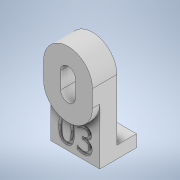
# Autodesk Inventor part: 1번부품
Saved by Autodesk Inventor 2022 (Build 260153000, 153)
## iProperties
Created: 2021-09-05
Part Number: 1번부품
Material: 일반
Document SubType Name: Modeling
Designer: 서울공업고등학교
Density: 1 g/cm^3
Appearance: 기본값
Author: 서울공업고등학교
Autodesk Inventor part; units mm, degrees
ref_plane "YZ Plane" through (0, 0, 0) normal (1, 0, 0) x (0, 1, 0)
ref_plane "XZ Plane" through (0, 0, 0) normal (0, 1, 0) x (-1, 0, 0)
ref_plane "XY Plane" through (0, 0, 0) normal (0, 0, 1) x (1, 0, 0)
sketch "스케치1" plane through (0, 0, 0) normal (0, 0, 1) x (1, 0, 0)
  line L0 (0, 0) -> (20, 0)
  line L1 (20, 0) -> (20, 40)
  line L2 (20, 40) -> (0, 40)
  line L3 (0, 40) -> (0, 0)
  line L4 (0, 13) -> (20, 13)
  line L5 (10, 30) -> (10, 23) construction
  line L6 (7, 30) -> (7, 23)
  line L7 (13, 23) -> (13, 30)
  arc A0 (13, 30) -> (7, 30) centre (10, 30) ccw
  arc A1 (7, 23) -> (13, 23) centre (10, 23) ccw
  point P0 (10, 26.5)
  dimension "d0" = 20
  dimension "d1" = 40
  dimension "d2" = 27
  dimension "d4" = 7
  dimension "d5" = 13.5
  dimension "d6" = 10
  dimension "d7" = 3
  constraints: 18 end point, 4 point on circle, 4 tangent, 3 parallel, 2 centre point, 2 perpendicular, 2 point on line, 1 horizontal, 1 midpoint, 1 vertical
  measures "d0" distance of L2.end L1.end
  measures "d1" distance of L1.end L0.end
  measures "d2" distance between parallel lines of L4 L2
  measures "d4" distance of L5.end L5.start
  measures "d5" distance from line of L2 point (10, 26.5)
  measures "d6" horizontal distance of L4.start L5.start
  measures "d7" radius of A1
extrude "돌출1" add sketch "스케치1" against normal blind 7
extrude "돌출2" add sketch "스케치1" along normal blind 3 contours L3 L2 L1 L4
fillet "모깎기1" radius 10 4 edges at (20, 40, -2) (0, 40, -2) (20, 13, 1.5) (0, 13, 1.5)
sketch "스케치2" plane through (0, 0, -7) normal (0, 0, -1) x (-1, 0, 0)
  line L0 (-20, 0) -> (-20, 23) projected
  line L1 (-20, 0) -> (0, 0) projected
  line L2 (-20, 0) -> (-20, 30) projected
  arc A0 (0, 30) -> (-20, 30) centre (-10, 30) ccw projected
  line L3 (0, 30) -> (0, 0) projected
  line L4 (0, 0) -> (-20, 0) projected
  line L5 (-13, 30) -> (-13, 23) projected
  arc A1 (-13, 23) -> (-7, 23) centre (-10, 23) ccw projected
  line L6 (-7, 23) -> (-7, 30) projected
  arc A2 (-7, 30) -> (-13, 30) centre (-10, 30) ccw projected
  line L7 (-20, 5) -> (0, 5)
  dimension "d14" = 5
  constraints: 2 end point, 2 point on line, 1 perpendicular
  measures "d14" distance between parallel lines of L1 L7
extrude "돌출3" add sketch "스케치2" along normal blind 8 contours L0 L7 L3 L1
sketch "스케치3" plane through (0, 0, 0) normal (0, 0, 1) x (1, 0, 0)
  line L0 (2.6578, 12.3276) -> (17.6998, 12.3276) construction
  line L1 (17.6998, 12.3276) -> (17.6998, 1.5834) construction
  line L2 (17.6998, 1.5834) -> (2.6578, 1.5834) construction
  line L3 (2.6578, 1.5834) -> (2.6578, 12.3276) construction
  spline S0 degree 2 poles (9.6108, 7.1169) (9.6108, 4.4265) (8.0468, 1.9062) (6.4179, 1.9062) knots 0 0 0 1 2 2 2
  spline S1 degree 2 poles (6.4179, 1.9062) (4.7648, 1.9062) (3.217, 4.4751) (3.217, 7.1088) knots 0 0 0 1 2 2 2
  spline S2 degree 2 poles (3.217, 7.1088) (3.217, 9.8155) (4.781, 12.3195) (6.4179, 12.3195) knots 0 0 0 1 2 2 2
  spline S3 degree 2 poles (6.4179, 12.3195) (8.063, 12.3195) (9.6108, 9.7263) (9.6108, 7.1169) knots 0 0 0 1 2 2 2
  spline S4 degree 2 poles (7.8928, 4.0699) (8.0873, 4.5643) (8.2494, 6.0878) (8.2494, 7.1169) knots 0 0 0 1 2 2 2
  spline S5 degree 2 poles (8.2494, 7.1169) (8.2494, 8.1461) (8.0873, 9.6615) (7.8847, 10.1721) knots 0 0 0 1 2 2 2
  spline S6 degree 2 poles (7.8847, 10.1721) (7.6821, 10.6826) (6.9771, 11.2093) (6.4179, 11.2093) knots 0 0 0 1 2 2 2
  spline S7 degree 2 poles (6.4179, 11.2093) (5.8588, 11.2093) (5.1375, 10.6826) (4.9268, 10.1558) knots 0 0 0 1 2 2 2
  spline S8 degree 2 poles (4.9268, 10.1558) (4.7242, 9.6453) (4.5784, 8.0894) (4.5784, 7.1088) knots 0 0 0 1 2 2 2
  spline S9 degree 2 poles (4.5784, 7.1088) (4.5784, 6.0554) (4.708, 4.6453) (4.9187, 4.0943) knots 0 0 0 1 2 2 2
  spline S10 degree 2 poles (4.9187, 4.0943) (5.1132, 3.5756) (5.8345, 3.0165) (6.4179, 3.0165) knots 0 0 0 1 2 2 2
  spline S11 degree 2 poles (6.4179, 3.0165) (6.969, 3.0165) (7.6902, 3.5432) (7.8928, 4.0699) knots 0 0 0 1 2 2 2
  spline S12 degree 2 poles (13.5897, 11.1688) (13.2251, 11.1688) (12.5038, 10.9905) (12.1554, 10.8528) knots 0 0 0 1 2 2 2
  spline S13 degree 2 poles (12.1554, 10.8528) (11.8312, 10.715) (11.3531, 10.4233) (11.1667, 10.2936) knots 0 0 0 1 2 2 2
  line L4 (11.1667, 10.2936) -> (11.0857, 10.2936)
  line L5 (11.0857, 10.2936) -> (11.0857, 11.7118)
  spline S14 degree 2 poles (11.0857, 11.7118) (11.5233, 11.9468) (13.0225, 12.3276) (13.6951, 12.3276) knots 0 0 0 1 2 2 2
  spline S15 degree 2 poles (13.6951, 12.3276) (14.3758, 12.3276) (15.3888, 12.0521) (15.802, 11.7604) knots 0 0 0 1 2 2 2
  spline S16 degree 2 poles (15.802, 11.7604) (16.2396, 11.4443) (16.6935, 10.5286) (16.6935, 9.9127) knots 0 0 0 1 2 2 2
  spline S17 degree 2 poles (16.6935, 9.9127) (16.6935, 9.0862) (15.6076, 7.8382) (14.8458, 7.6761) knots 0 0 0 1 2 2 2
  line L6 (14.8458, 7.6761) -> (14.8458, 7.5789)
  spline S18 degree 2 poles (14.8458, 7.5789) (15.1618, 7.514) (15.8831, 7.2223) (16.191, 6.9306) knots 0 0 0 1 2 2 2
  spline S19 degree 2 poles (16.191, 6.9306) (16.499, 6.6469) (16.8879, 5.7393) (16.8879, 5.0829) knots 0 0 0 1 2 2 2
  spline S20 degree 2 poles (16.8879, 5.0829) (16.8879, 4.4103) (16.426, 3.2677) (16.0046, 2.8301) knots 0 0 0 1 2 2 2
  spline S21 degree 2 poles (16.0046, 2.8301) (15.567, 2.3763) (14.3272, 1.9062) (13.5411, 1.9062) knots 0 0 0 1 2 2 2
  spline S22 degree 2 poles (13.5411, 1.9062) (12.7875, 1.9062) (11.3126, 2.2709) (10.8101, 2.5221) knots 0 0 0 1 2 2 2
  line L7 (10.8101, 2.5221) -> (10.8101, 3.9403)
  line L8 (10.8101, 3.9403) -> (10.9074, 3.9403)
  spline S23 degree 2 poles (10.9074, 3.9403) (11.3288, 3.6323) (12.755, 3.0651) (13.4601, 3.0651) knots 0 0 0 1 2 2 2
  spline S24 degree 2 poles (13.4601, 3.0651) (13.8734, 3.0651) (14.6999, 3.3244) (14.9755, 3.6242) knots 0 0 0 1 2 2 2
  spline S25 degree 2 poles (14.9755, 3.6242) (15.2429, 3.9241) (15.5265, 4.6372) (15.5265, 5.1802) knots 0 0 0 1 2 2 2
  spline S26 degree 2 poles (15.5265, 5.1802) (15.5265, 5.7231) (15.2105, 6.4281) (14.9268, 6.6307) knots 0 0 0 1 2 2 2
  spline S27 degree 2 poles (14.9268, 6.6307) (14.6432, 6.8333) (13.8734, 6.9873) (13.4195, 6.9873) knots 0 0 0 1 2 2 2
  line L9 (13.4195, 6.9873) -> (12.8523, 6.9873)
  line L10 (12.8523, 6.9873) -> (12.8523, 8.0975)
  line L11 (12.8523, 8.0975) -> (13.298, 8.0975)
  spline S28 degree 2 poles (13.298, 8.0975) (14.1975, 8.0975) (15.332, 8.9565) (15.332, 9.775) knots 0 0 0 1 2 2 2
  spline S29 degree 2 poles (15.332, 9.775) (15.332, 10.1558) (15.0403, 10.6988) (14.8053, 10.8609) knots 0 0 0 1 2 2 2
  spline S30 degree 2 poles (14.8053, 10.8609) (14.5541, 11.031) (13.9382, 11.1688) (13.5897, 11.1688) knots 0 0 0 1 2 2 2
  point P0 (0, 0)
  constraints: 2 other
extrude "돌출4" cut sketch "스케치3" against normal blind 1
